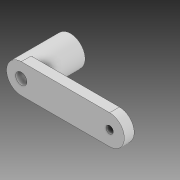
# Autodesk Inventor part: ServoArm
Saved by Autodesk Inventor 2020 (Build 240168000, 168)
## iProperties
Created: 2021-05-14
Part Number: ServoArm
Material: Generic
Document SubType Name: Modeling
Designer: DDeGo
Density: 1 g/cm^3
Appearance: Default
Author: DDeGo
Autodesk Inventor part; units mm, degrees
ref_plane "YZ Plane" through (0, 0, 0) normal (1, 0, 0) x (0, 1, 0)
ref_plane "XZ Plane" through (0, 0, 0) normal (0, 1, 0) x (-1, 0, 0)
ref_plane "XY Plane" through (0, 0, 0) normal (0, 0, 1) x (1, 0, 0)
sketch "Sketch1" plane through (0, 0, 0) normal (0, 0, 1) x (1, 0, 0)
  circle A0 centre (0, 0) radius 1.15
  line L0 (0, 0) -> (18, 0) construction
  line L1 (0, -3) -> (18, -3)
  line L2 (18, 3) -> (0, 3)
  arc A1 (0, 3) -> (0, -3) centre (0, 0) ccw
  arc A2 (18, -3) -> (18, 3) centre (18, 0) ccw
  circle A3 centre (18, 0) radius 0.75
  point P0 (9, 0)
  dimension "d0" = 2.3
  dimension "d1" = 3
  dimension "d2" = 1.5
  dimension "d3" = 18
  constraints: 8 end point, 4 centre point, 4 point on circle, 4 tangent, 2 coincident, 1 horizontal, 1 midpoint, 1 parallel
  measures "d0" diameter of A0
  measures "d1" radius of A1
  measures "d2" diameter of A3
  measures "d3" distance of L0.start L0.end
extrude "Extrusion1" add sketch "Sketch1" along normal blind 2
sketch "Sketch2" plane through (0, 0, 0) normal (0, 0, -1) x (-1, 0, 0)
  arc A0 (0, -3) -> (0, 3) centre (0, 0) ccw projected
  circle A1 centre (0, 0) radius 3
  circle A2 centre (0, 0) radius 1.15
  circle A3 centre (0, 0) radius 1.15 projected
  point P0 (0, -3)
  constraints: 2 coincident, 1 centre point, 1 concentric, 3 other
extrude "Extrusion2" add sketch "Sketch2" along normal blind 8
body "Solid1"
